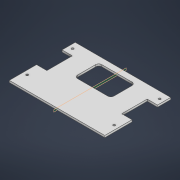
# Autodesk Inventor part: old
Saved by Autodesk Inventor 2022 (Build 260153000, 153)
## iProperties
Created: 2022-01-27
Part Number: old
Material: 一般
Document SubType Name: Sheet Metal
Designer: shiokaze
Density: 1 g/cm^3
Sheet Metal Rule: Default_mm
Appearance: 既定
Author: shiokaze
Autodesk Inventor part; units mm, degrees
ref_plane "YZ Plane" through (0, 0, 0) normal (1, 0, 0) x (0, 1, 0)
ref_plane "XZ Plane" through (0, 0, 0) normal (0, 1, 0) x (-1, 0, 0)
ref_plane "XY Plane" through (0, 0, 0) normal (0, 0, 1) x (1, 0, 0)
sketch "スケッチ1" plane through (0, 0, 0) normal (0, 1, 0) x (-1, 0, 0)
  line L0 (39.4, -27.2) -> (0, -27.2)
  line L1 (0, -27.2) -> (0, 27.2)
  line L2 (0, 27.2) -> (39.4, 27.2)
  line L3 (39.4, -16.3) -> (30.9, -16.3)
  line L4 (30.9, -16.3) -> (30.9, 4.7)
  line L5 (30.9, 4.7) -> (39.4, 4.7)
  line L6 (39.4, 4.7) -> (39.4, -16.3) construction
  line L7 (39.4, 27.2) -> (39.4, 4.7)
  line L8 (39.4, -16.3) -> (39.4, -27.2)
  point P0 (0, 0)
  point P1 (0, 0)
  dimension "d0" = 10.9
  dimension "d1" = 22.5
  dimension "d2" = 39.4
  dimension "d3" = 21
  dimension "d5" = 8.5
  constraints: 18 end point, 5 parallel, 2 collinear, 2 horizontal, 2 perpendicular, 1 coincident, 1 midpoint
  measures "d0" distance between parallel lines of L0 L3
  measures "d1" distance between parallel lines of L2 L5
  measures "d2" distance of L1.end L2.end
  measures "d3" distance of L5.end L3.start
  measures "d5" distance between parallel lines of L4 L6
extrude "押し出し1" add sketch "スケッチ1" along normal blind 1.6
sketch "スケッチ2" plane through (0, 1.6, 0) normal (0, 1, 0) x (1, 0, 0)
  line L0 (-30.9, 16.3) -> (-30.9, -4.7) projected
  line L1 (-30.9, -4.7) -> (-39.4, -4.7) projected
  line L2 (-39.4, -4.7) -> (-39.4, -27.2) projected
  line L3 (-39.4, -27.2) -> (0, -27.2) projected
  line L4 (0, -27.2) -> (0, 27.2) projected
  line L5 (0, 27.2) -> (-39.4, 27.2) projected
  line L6 (-39.4, 27.2) -> (-39.4, 16.3) projected
  line L7 (-39.4, 16.3) -> (-30.9, 16.3) projected
  point P0 (0, 0)
  point P1 (-35.9, 21.55)
  point P2 (-35.9, -15.95)
  dimension "d8" = 11.25
  dimension "d9" = 5.25
  dimension "d10" = 3.5
  dimension "d11" = 3.5
  measures "d8" distance from line of L1 point (-35.9, -15.95)
  measures "d9" distance from line of L7 point (-35.9, 21.55)
  measures "d10" distance from line of L6 point (-35.9, 21.55)
  measures "d11" distance from line of L2 point (-35.9, -15.95)
hole "穴1" at (-35.9, 1.6, -21.55) at (-35.9, 1.6, 15.95) direction (0, -1, 0) diameter 1.8 end through all
mirror "ミラー1" about plane through (0, 0, 27.2) normal (1, 0, 0) of "押し出し1"
ref_plane "作業平面1" through (0, 0, 4.7) normal (-1, 0, 0) x (0, 0, 1)
mirror "ミラー2" about plane through (0, 0, 4.7) normal (-1, 0, 0) of "穴1", "押し出し1"
sketch "スケッチ3" plane through (0, 1.6, 0) normal (0, 1, 0) x (1, 0, 0)
  circle A0 centre (35.9, 21.55) radius 0.9 projected
  circle A1 centre (35.9, -15.95) radius 0.9 projected
  line L0 (-39.4, 27.2) -> (39.4, 27.2) projected
  line L1 (-39.4, 27.2) -> (-39.4, 16.3) projected
  line L2 (-39.4, 16.3) -> (-30.9, 16.3) projected
  line L3 (-30.9, 16.3) -> (-30.9, -4.7) projected
  line L4 (-30.9, -4.7) -> (-39.4, -4.7) projected
  line L5 (-39.4, -4.7) -> (-39.4, -27.2) projected
  line L6 (-39.4, -27.2) -> (39.4, -27.2) projected
  line L7 (39.4, -4.7) -> (39.4, -27.2) projected
  line L8 (30.9, -4.7) -> (39.4, -4.7) projected
  line L9 (30.9, 16.3) -> (30.9, -4.7) projected
  line L10 (39.4, 16.3) -> (30.9, 16.3) projected
  line L11 (39.4, 27.2) -> (39.4, 16.3) projected
  circle A2 centre (-35.9, 21.55) radius 0.9 projected
  circle A3 centre (-35.9, -15.95) radius 0.9 projected
  line L12 (-15, 22.2) -> (0, 22.2)
  line L13 (0, 22.2) -> (0, 2.2)
  line L14 (0, 2.2) -> (-15, 2.2)
  line L15 (-15, 2.2) -> (-15, 22.2)
  line L16 (15, 22.2) -> (0, 22.2)
  line L17 (0, 2.2) -> (15, 2.2)
  line L18 (15, 2.2) -> (15, 22.2)
  line L19 (-39.4, 16.3) -> (-30.9, 16.3) projected
  line L20 (-30.9, 16.3) -> (-30.9, -4.7)
  line L21 (30.9, 16.3) -> (30.9, -4.7) projected
  line L22 (30.9, -4.7) -> (30.9, 16.3)
  line L23 (-30.9, 16.3) -> (-30.9, -4.7) projected
  point P0 (0, 0)
  point P1 (0, 12.2)
  dimension "d19" = 30
  dimension "d21" = 20
  dimension "d26" = 5
  dimension "d28" = 39.4
  constraints: 18 end point, 3 equal length, 2 symmetric about line, 1 horizontal, 1 midpoint, 1 perpendicular, 1 vertical
  measures "d19" distance between parallel lines of L18 L15
  measures "d21" distance of L14.end L12.start
  measures "d26" distance between parallel lines of L0 L12
  measures "d28" distance between parallel lines of L1 L13
extrude "押し出し2" cut sketch "スケッチ3" against normal blind 10 contours L12 L13 L14 L15 | L16 L18 L17 L13
fillet "フィレット1" radius 2.5 4 edges at (-15, 0.8, -22.2) (-15, 0.8, -2.2) (15, 0.8, -2.2) (15, 0.8, -22.2)
equation "\"d17\" = Thickness"
equation "\"BendRadius\" = Thickness"
equation "\"BendReliefWidth\" = Thickness"
equation "\"BendReliefDepth\" = 0.5 * Thickness"
equation "\"CornerReliefSize\" = 4 * Thickness"
equation "\"MinimumRemnant\" = 2 * Thickness"
equation "\"TransitionRadius\" = BendRadius"
equation "\"JacobiRadiusSize\" = BendRadius"
equation "\"GapSize\" = Thickness"
equation "\"Thickness\" = 0.5"
